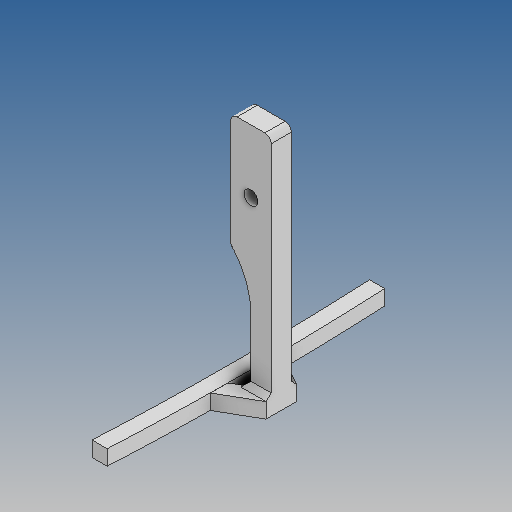
# Autodesk Inventor part: Gripper neu
Saved by Autodesk Inventor 2026.2 (Build 302298000, 298)
## iProperties
Created: 2025-12-08
Part Number: Gripper neu
Material: Generisch
Document SubType Name: Modeling
Designer: Schally
Density: 1 g/cm^3
Appearance: Vorgabe
Author: Schally
Autodesk Inventor part; units mm, degrees
ref_plane "YZ Plane" through (0, 0, 0) normal (1, 0, 0) x (0, 1, 0)
ref_plane "XZ Plane" through (0, 0, 0) normal (0, 1, 0) x (-1, 0, 0)
ref_plane "XY Plane" through (0, 0, 0) normal (0, 0, 1) x (1, 0, 0)
sketch "Skizze2" plane through (0, 0, 0) normal (0, 0, 1) x (1, 0, 0)
  line L0 (-45.7004, 0) -> (8.2208, 0) projected
  line L1 (0, -18.1036) -> (0, 108.6213) projected
  circle A0 centre (-8, 65) radius 2.7
  line L2 (0, 0) -> (0, 87.5)
  arc A1 (0, 87.5) -> (-2.5, 90) centre (-2.5, 87.5) ccw
  line L3 (-13.5, 90) -> (-2.5, 90)
  arc A2 (-13.5, 90) -> (-16, 87.5) centre (-13.5, 87.5) ccw
  line L4 (-16, 87.5) -> (-16, 45)
  line L5 (-8, 0) -> (-8, 25)
  line L6 (0, 0) -> (-8, 0)
  arc A3 (-8, 25) -> (-16, 45) centre (-37.9973, 24.6011) ccw
  point P0 (0, 0)
  point P1 (-4, 0)
  dimension "d0" = 90
  dimension "d1" = 8
  dimension "d2" = 16
  dimension "d4" = 2.5
  dimension "d5" = 2.5
  dimension "d6" = 5.4
  dimension "d8" = 25
  dimension "d11" = 25
  dimension "d16" = 2.5
  dimension "d17" = 2.5
  dimension "d18" = 2.5
  dimension "d19" = 2.5
  dimension "d90" = 45
  dimension "d126" = 30
  dimension "d131" = 40
  dimension "d132" = 8
  constraints: 10 end point, 6 point on circle, 4 centre point, 1 coincident, 1 horizontal alignment, 1 midpoint, 1 parallel, 1 vertical
  measures "d0" distance between parallel lines of L6 L3
  measures "d1" distance between parallel lines of L5 L2
  measures "d2" distance between parallel lines of L2 L4
  measures "d4" radius of A1
  measures "d5" radius of A2
  measures "d6" diameter of A0
  measures "d8" distance from line of L3 A0.centre
  measures "d11" distance from line of L6 L5.end
  measures "d16" distance from line of L4 A2.centre
  measures "d17" distance from line of A2.centre L3
  measures "d18" distance from line of A1.centre L3
  measures "d19" distance from line of A1.centre L1
  measures "d90" distance from line of L4.end L3
  measures "d126" radius of A3
  measures "d131" distance of L5.end A0.centre
  measures "d132" distance from line of A0.centre L4
extrude "Extrusion1" add sketch "Skizze2" along normal mid plane 8
sketch "Skizze5" plane through (-8, 0, 4) normal (0, -1, 0) x (1, 0, 0)
  line L0 (8, -8) -> (8, 0) projected
  line L1 (0, 0) -> (8, 0) projected
  line L2 (0, -8) -> (0, 0) projected
  line L3 (8, -8) -> (0, -8) projected
  line L4 (-2, -10) -> (-2, 2)
  line L5 (-2, 2) -> (10, 2)
  line L6 (10, 2) -> (10, -10)
  line L7 (10, -10) -> (-2, -10)
  line L8 (8, -10) -> (8, 2)
  line L9 (8, -10) -> (-6, -18.0829)
  line L10 (8, -10) -> (48, -10) construction
  line L11 (8, 2) -> (-6, 10.0829)
  line L12 (8, 2) -> (48, 2) construction
  line L13 (-6, 26.9678) -> (-6, -33.1167)
  line L14 (-2, 0.8453) -> (-6, 3.1547)
  line L15 (-6, -11.1547) -> (-2, -8.8453)
  point P0 (8, -4)
  dimension "d103" = 2
  dimension "d104" = 150
  dimension "d107" = 150
  dimension "d108" = 6
  dimension "d113" = 6
  dimension "d114" = 6
  constraints: 24 end point, 9 point on line, 2 horizontal, 2 vertical, 3 other
  measures "d103" distance between parallel lines of L3 L7
  measures "d104" angle of L9 L10
  measures "d107" angle of L12 L11
  measures "d108" distance between parallel lines of L13 L2
  measures "d113" distance between parallel lines of L11 L14
  measures "d114" distance between parallel lines of L9 L15
extrude "Extrusion3" add sketch "Skizze5" along normal blind 6 contours L3 L2 L1 L0 | L8 L7 L4 L5 L1 L2 L3 | L9 L13 L15 L4 L7 | L5 L4 L14 L13 L11
sketch "Skizze6" plane through (-14, 0, -14.0829) normal (-1, 0, 0) x (0, 0, 1)
  arc A0 (-91.4171, 6.8936) -> (119.5829, 6.8936) centre (14.0829, 1117.4186) ccw
  line L0 (14.0829, 1343.255) -> (14.0829, -237.5996) projected
  line L1 (-134.6641, 0) -> (162.8299, 0) projected
  line L2 (6.9282, 0) -> (0, 0) projected
  line L3 (0, 0) -> (0, -6) projected
  line L4 (6.9282, -6) -> (0, -6) projected
  line L5 (6.9282, 0) -> (6.9282, -6) projected
  line L6 (28.1658, 0) -> (21.2376, 0) projected
  line L7 (21.2376, 0) -> (21.2376, -6) projected
  line L8 (28.1658, -6) -> (21.2376, -6) projected
  line L9 (28.1658, 0) -> (28.1658, -6) projected
  line L10 (69.0829, 4.8846) -> (69.0829, -11.7632)
  line L11 (-40.9171, 6.8936) -> (-40.9171, -11.0991)
  arc A1 (-40.9171, 1.3407) -> (69.0829, 1.3407) centre (14.0829, 1117.4186) ccw
  arc A2 (-92.1649, -0.9783) -> (120.3307, -0.9783) centre (14.0829, 1117.4186) ccw
  point P0 (14.0829, 0)
  point P1 (-40.9171, 0.6181)
  point P2 (69.0829, -4.6666)
  point P3 (69.0829, 0.908)
  point P4 (-40.9171, 1.6575)
  point P5 (-40.9171, -4.6666)
  dimension "d122" = 6
  dimension "d127" = 110
  constraints: 6 point on circle, 4 end point, 4 point on line, 3 centre point, 2 horizontal alignment, 2 vertical, 1 other
  measures "d122" radial gap between concentric circles of A1 A2
  measures "d127" distance between parallel lines of L10 L11
extrude "Extrusion4" add sketch "Skizze6" along normal blind 6 contours A1 L1 L11 | L1 L3 A2 L11 | A1 L0 A2 L5 L1 | L10 L1 A1 | A1 L1 L7 A2 L0 | L1 L5 A2 L3 | L10 A2 L9 L1 | L1 L9 A2 L7
chamfer "Fasen6" distance 2 angle 45 3 edges at (-4, 0, -4) (-8, 0, 0) (-4, 0, 4)
fillet "Rundung1" radius 2 1 edges at (-16, 45, 0)
sketch "Skizze7" plane through (0, 0, -4) normal (0, 0, -1) x (-1, 0, 0)
  arc A0 (15.4998, 44.447) -> (16, 45.7701) centre (14, 45.7701) ccw projected
  line L0 (16, 45.7701) -> (16, 87.5) projected
  arc A1 (16, 87.5) -> (13.5, 90) centre (13.5, 87.5) ccw projected
  line L1 (13.5, 90) -> (2.5, 90) projected
  arc A2 (2.5, 90) -> (0, 87.5) centre (2.5, 87.5) ccw projected
  line L2 (0, 87.5) -> (0, 2) projected
  line L3 (8, 2) -> (0, 2) projected
  line L4 (8, 2) -> (8, 25) projected
  arc A3 (15.4998, 44.447) -> (8, 25) centre (37.9973, 24.6011) ccw projected
  circle A4 centre (8, 65) radius 2.7 projected
  circle A5 centre (8, 65) radius 6.5
  line L5 (8, 85) -> (8, 45)
  line L6 (12.5, 82.2483) -> (12.5, 48.2483)
  line L7 (3.5, 48.5932) -> (3.5, 82.5932)
  circle A6 centre (8, 82) radius 3
  circle A7 centre (8, 48) radius 3
  line L8 (17.259, 81.9916) -> (-1.9844, 81.9916)
  line L9 (19.4429, 48.0084) -> (-6.0611, 48.0084)
  line L10 (5, 48.0084) -> (3.5, 60.3096)
  line L11 (11, 48.0084) -> (12.5, 60.3096)
  line L12 (3.5, 69.6904) -> (5, 81.9929)
  line L13 (12.5, 69.6904) -> (10.4193, 81.9916)
  point P0 (0, 0)
  point P1 (10.6543, 80.602)
  dimension "d142" = 6
  dimension "d133" = 13
  dimension "d136" = 20
  dimension "d137" = 20
  dimension "d143" = 3
  dimension "d144" = 6
  dimension "d145" = 3
  dimension "d146" = 9
  constraints: 18 end point, 9 point on line, 6 point on circle, 2 centre point, 1 coincident, 1 vertical, 1 vertical alignment, 4 other
  measures "d133" diameter of A5
  measures "d136" distance of A4.centre L5.start
  measures "d137" distance of L5.end A4.centre
  measures "d143" distance of point (8, 82) L5.start
  measures "d144" diameter of A7
  measures "d145" distance of L5.end A7.centre
  measures "d146" distance between parallel lines of L6 L7
extrude "Extrusion5" cut sketch "Skizze7" against normal blind 4 contours L9 L5 A7 | A7 L5 L9 | A7 L5 A5 L11 | A7 L10 A5 L5 | L5 L9 A7 | L5 A7 L9 | L6 A5 | A5 L5 A4 L6 | A5 L5 A6 L13 | L8 L5 A6 | A6 L13 L8 | A5 L7 L5 A4 | A5 L12 A6 L5 | A6 L5 L8 L13 | A5 L7 | A6 L8 L5 | L5 L8 A6
